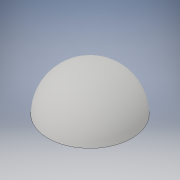
# Autodesk Inventor part: HighvLowResTest
Saved by Autodesk Inventor 2018 (Build 220112000, 112)
## iProperties
Created: 2019-09-03
Part Number: HighvLowResTest
Material: Generic
Document SubType Name: Modeling
Designer: 871357
Density: 1 g/cm^3
Appearance: Default
Author: 871357
Autodesk Inventor part; units mm, degrees
ref_plane "YZ Plane" through (0, 0, 0) normal (1, 0, 0) x (0, 1, 0)
ref_plane "XZ Plane" through (0, 0, 0) normal (0, 1, 0) x (-1, 0, 0)
ref_plane "XY Plane" through (0, 0, 0) normal (0, 0, 1) x (1, 0, 0)
sketch "Sketch1" plane through (0, 0, 0) normal (0, 0, 1) x (1, 0, 0)
  arc A0 (6.35, 0) -> (-6.35, 0) centre (0, 0) ccw
  line L0 (-6.35, 0) -> (6.35, 0)
  dimension "d0" = 12.7
  constraints: 2 end point, 2 point on circle, 1 centre point, 1 coincident, 1 horizontal
  measures "d0" diameter of A0
revolve "Revolution1" add sketch "Sketch1" angle 180 mid plane about axis through (-6.35, 0, 0) along (1, 0, 0)
body "Solid1"
